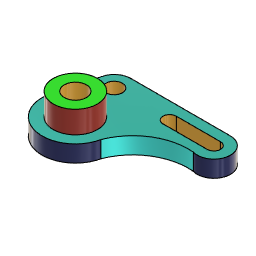
Ex 4 v3 (Autodesk Fusion 360 design; units mm, degrees)
Autodesk Fusion 360 part; units mm, degrees
sketch "Sketch1" plane through (0, 0, 0) normal (0, 0, 1) x (1, 0, 0)
  circle A0 centre (0, 0) radius 10
  circle A1 centre (0, 0) radius 20
  line L0 (44.8684, 45.9986) -> (85.1316, 45.9986)
  line L1 (44.8684, 34.0014) -> (85.0003, 34)
  arc A2 (45.1316, 45.9986) -> (45.1312, 34.0014) centre (45, 40) ccw
  arc A3 (80.8572, 25.5834) -> (84.8684, 54.9994) centre (85, 40) ccw
  arc A4 (84.9992, 34) -> (84.8684, 45.9986) centre (85, 40) ccw
  line L2 (84.8684, 54.9994) -> (-5.1316, 54.9994)
  circle A5 centre (-5, 40) radius 7.5
  arc A6 (-4.8019, 54.9994) -> (-19.5455, 43.5305) centre (-4.9668, 40.0003) ccw
  line L3 (-28.779, 8.4716) -> (-19.393, 44.1092)
  arc A7 (80.8572, 25.5834) -> (29.3388, -6.2637) centre (76.0178, -24.1816) ccw
  arc A8 (-28.779, 8.4716) -> (29.3388, -6.2637) centre (0, 0) ccw
  constraint coincident A0.centre A1.centre
  constraint concentric A3 A4
  constraint coincident L0.start A2
  constraint coincident L0.end A4
  constraint horizontal L0
  constraint coincident L1.start A2
  constraint coincident L1.end A4
  constraint coincident L0 A2.start
  constraint coincident L1 A2.end
  constraint coincident L0 A4.end
  constraint coincident L1 A4.start
  constraint parallel L0 L2
  constraint coincident L2.end A6
  constraint coincident L2 A6.start
  constraint coincident L3 A6.end
  constraint coincident A6 L3.end
sketch "Sketch2" plane through (0, 0, 0) normal (0, 0, 1) x (1, 0, 0)
extrude "Extrude1" add sketch "Sketch1" along normal blind 15 contours A3 L2 A6 L3 A7 A8
extrude "Extrude2" add sketch "Sketch1" along normal blind 35 contours A1
